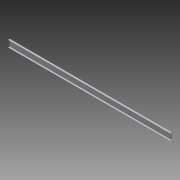
# Autodesk Inventor part: channel2.25x4
Saved by Autodesk Inventor 2013 (Build 170138000, 138)
## iProperties
Created: 2013-01-31
Part Number: channel2.25x4
Material: Aluminum 6061
Document SubType Name: Modeling
Designer: istvan.burbank
Density: 1 g/cm^3
Author: istvan.burbank
Autodesk Inventor part; units mm, degrees
ref_plane "YZ Plane" through (0, 0, 0) normal (1, 0, 0) x (0, 1, 0)
ref_plane "XZ Plane" through (0, 0, 0) normal (0, 1, 0) x (-1, 0, 0)
ref_plane "XY Plane" through (0, 0, 0) normal (0, 0, 1) x (1, 0, 0)
sketch "Sketch1" plane through (0, 0, 0) normal (1, 0, 0) x (0, 1, 0)
  line L0 (0, 0) -> (101.6, 0)
  line L1 (101.6, 0) -> (101.6, 25.4)
  line L2 (0, 25.4) -> (0, 0)
  line L3 (98.425, 25.4) -> (98.425, 3.175)
  line L4 (98.425, 3.175) -> (3.175, 3.175)
  line L5 (3.175, 3.175) -> (3.175, 25.4)
  line L6 (101.6, 25.4) -> (98.425, 25.4)
  line L7 (3.175, 25.4) -> (0, 25.4)
  dimension "d0" = 101.6
  dimension "d1" = 25.4
  dimension "d2" = 3.175
  constraints: 18 end point, 4 parallel, 2 perpendicular, 1 collinear, 1 horizontal, 2 other
  measures "d0" distance of L2.start L1.end
  measures "d1" distance of L1.end L0.end
  measures "d2" distance between parallel lines of L0 L4
extrude "Extrusion1" add sketch "Sketch1" against normal blind 2438.4
body "Solid1"
